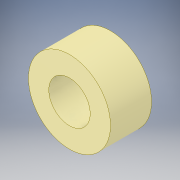
# Autodesk Inventor part: Spacer_Round_0.5x0.5
Saved by Autodesk Inventor 2017 (Build 210142000, 142)
## iProperties
Created: 2017-01-29
Part Number: Spacer_Round_0.5x0.5
Material: Nylon 6/6
Document SubType Name: Modeling
Designer: Beezy
Density: 1.13 g/cm^3
Appearance: Nylon 6
Author: Beezy
Autodesk Inventor part; units mm, degrees
ref_plane "YZ Plane" through (0, 0, 0) normal (1, 0, 0) x (0, 1, 0)
ref_plane "XZ Plane" through (0, 0, 0) normal (0, 1, 0) x (-1, 0, 0)
ref_plane "XY Plane" through (0, 0, 0) normal (0, 0, 1) x (1, 0, 0)
sketch "Sketch1" plane through (0, 0, 0) normal (0, 0, 1) x (1, 0, 0)
  circle A0 centre (0, 0) radius 6.4135
  circle A1 centre (0, 0) radius 12.7
  dimension "d0" = 12.827
  dimension "d1" = 25.4
  constraints: 2 centre point, 2 coincident
  measures "d0" diameter of A0
  measures "d1" diameter of A1
extrude "Extrusion1" add sketch "Sketch1" against normal blind 12.7
body "Solid1"
